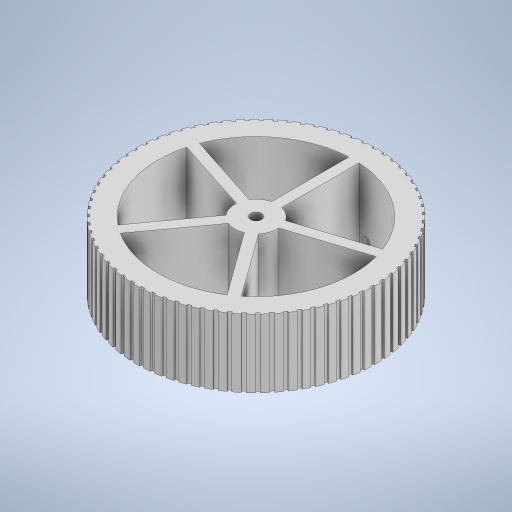
# Autodesk Inventor part: wheel
Saved by Autodesk Inventor 2023 (Build 270158000, 158)
## iProperties
Created: 2022-10-31
Part Number: wheel
Material: Generic
Document SubType Name: Modeling
Designer: neera
Density: 1 g/cm^3
Appearance: Default
Author: neera
Autodesk Inventor part; units mm, degrees
ref_plane "YZ Plane" through (0, 0, 0) normal (1, 0, 0) x (0, 1, 0)
ref_plane "XZ Plane" through (0, 0, 0) normal (0, 1, 0) x (-1, 0, 0)
ref_plane "XY Plane" through (0, 0, 0) normal (0, 0, 1) x (1, 0, 0)
sketch "Sketch1" plane through (0, 0, 0) normal (0, 1, 0) x (-1, 0, 0)
  circle A0 centre (0, 0) radius 70
  dimension "d0" = 140
  constraints: 1 centre point, 1 coincident
  measures "d0" diameter of A0
extrude "Extrusion1" add sketch "Sketch1" along normal blind 40
sketch "Sketch3" plane through (0, 40, 0) normal (0, 1, 0) x (1, 0, 0)
  circle A0 centre (0, 0) radius 57.5
  line L0 (0, 0) -> (57.5, 0) construction
  circle A1 centre (0, 0) radius 12.5
  line L1 (3, 12.1347) -> (3, 57.4217)
  line L2 (-3, 12.1347) -> (-3, 57.4217)
  line L3 (-10.6137, 6.603) -> (-53.6842, 20.5974)
  line L4 (-12.4678, 0.8966) -> (-55.5383, 14.8911)
  line L5 (-9.5596, -8.0538) -> (-36.1787, -44.6918)
  line L6 (-4.7055, -11.5805) -> (-31.3246, -48.2185)
  line L7 (4.7055, -11.5805) -> (31.3246, -48.2185)
  line L8 (9.5596, -8.0538) -> (36.1787, -44.6918)
  line L9 (12.4678, 0.8966) -> (55.5383, 14.8911)
  line L10 (10.6137, 6.603) -> (53.6842, 20.5974)
  point P0 (53.6842, 20.5974)
  dimension "d6" = 115
  dimension "d8" = 25
  dimension "d9" = 3
  dimension "d10" = 3
  dimension "d13" = 360
  constraints: 22 end point, 4 point on circle, 2 centre point, 2 coincident, 2 vertical, 1 horizontal, 31 other
  measures "d6" diameter of A0
  measures "d8" diameter of A1
  measures "d9" horizontal distance of point (0, 0) L1.start
  measures "d10" horizontal distance of point (0, 0) L2.start
extrude "Extrusion3" cut sketch "Sketch3" against normal blind 40 contours A0 L8 A1 L9 | L10 A1 L1 A0 | A0 L6 A1 L7 | L2 A1 L3 A0 | A0 L4 A1 L5
sketch "Sketch5" plane through (0, 0, 0) normal (0, -1, 0) x (1, 0, 0)
  arc A0 (-3.15, 0) -> (3.15, 0) centre (0, 0) ccw
  line L0 (3.15, 0) -> (12.5, 0)
  arc A1 (12.4678, -0.8966) -> (9.5596, 8.0538) centre (0, 0) ccw projected
  arc A2 (-1.695, 2.6551) -> (1.695, 2.6551) centre (0, 0) ccw projected
  line L1 (-3.15, 0) -> (-12.5073, 0)
  arc A3 (-12.5073, 0) -> (12.5, 0) centre (-0.0036, 0) ccw
  constraints: 6 point on circle, 4 end point, 2 centre point, 2 point on line, 1 coincident, 1 horizontal
extrude "Extrusion5" cut sketch "Sketch5" against normal blind 5
sketch "Sketch6" plane through (0, 0, 0) normal (0, -1, 0) x (1, 0, 0)
  circle A0 centre (0, 0) radius 3.15
  constraints: 1 centre point, 1 coincident
extrude "Extrusion6" cut sketch "Sketch6" against normal blind 40
sketch "Sketch7" plane through (12.5, 0, 0) normal (0, 0, -1) x (-1, 0, 0)
  circle A0 centre (4.675, 2.5) radius 1.5
  line L0 (9.35, 0) -> (9.35, 5) projected
  circle A1 centre (20.325, 2.5) radius 1.5
  line L1 (15.65, 0) -> (15.65, 5) projected
  line L2 (25, 5) -> (15.65, 5) projected
  line L3 (9.35, 5) -> (0, 5) projected
  point P0 (12.5, 0)
  point P1 (9.35, 2.5)
  point P2 (15.65, 2.5)
  point P3 (20.325, 5)
  point P4 (4.675, 5)
  dimension "d25" = 3
  dimension "d26" = 4.675
  dimension "d27" = 3
  dimension "d28" = 4.675
  dimension "d29" = 2.5
  dimension "d30" = 2.5
  constraints: 4 midpoint, 2 centre point
  measures "d25" diameter of A0
  measures "d26" distance of point (9.35, 2.5) A0.centre
  measures "d27" diameter of A1
  measures "d28" distance of point (15.65, 2.5) A1.centre
  measures "d29" distance of point (20.325, 5) A1.centre
  measures "d30" distance of point (4.675, 5) A0.centre
extrude "Extrusion7" cut sketch "Sketch7" against normal blind 4.5
sketch "Sketch8" plane through (0, 0, 0) normal (0, -1, 0) x (1, 0, 0)
  line L0 (6.325, 0) -> (6.325, 4.5) projected
  line L1 (9.325, 0) -> (9.325, 4.5) projected
  line L2 (6.325, 3) -> (9.325, 3)
  line L3 (9.325, 3) -> (9.325, 4.5)
  line L4 (9.325, 4.5) -> (6.325, 4.5)
  line L5 (6.325, 4.5) -> (6.325, 3)
  line L6 (-9.325, 0) -> (-9.325, 4.5) projected
  line L7 (-6.325, 0) -> (-6.325, 4.5) projected
  line L8 (-9.325, 3) -> (-6.325, 3)
  line L9 (-6.325, 3) -> (-6.325, 4.5)
  line L10 (-6.325, 4.5) -> (-9.325, 4.5)
  line L11 (-9.325, 4.5) -> (-9.325, 3)
  line L12 (-12.5, 0) -> (-3.15, 0) projected
  line L13 (3.15, 0) -> (12.5, 0) projected
  point P0 (0, 0)
  point P1 (-7.825, 0)
  point P2 (-7.825, 3)
  point P3 (7.825, 0)
  point P4 (7.825, 4.5)
  dimension "d33" = 3
  dimension "d34" = 4.5
  constraints: 16 end point, 6 point on line, 4 midpoint, 4 parallel, 2 horizontal, 2 perpendicular
  measures "d33" distance of point (-7.825, 0) point (-7.825, 3)
  measures "d34" distance of point (7.825, 0) point (7.825, 4.5)
extrude "Extrusion8" cut sketch "Sketch8" against normal blind 6 contours L0 L4 L1 L2 | L6 L10 L7 L8
sketch "Sketch9" plane through (0, 0, 0) normal (0, -1, 0) x (1, 0, 0)
  line L0 (1, -71) -> (-1, -71)
  line L1 (-1, -71) -> (-1, -69)
  line L2 (-1, -69) -> (1, -69)
  line L3 (1, -69) -> (1, -71)
  circle A0 centre (0, 0) radius 70 projected
  line L4 (1, -71) -> (-1, -69) construction
  line L5 (-1, -71) -> (1, -69) construction
  line L6 (4.7773, -68.8417) -> (6.7703, -68.6743)
  line L7 (6.7703, -68.6743) -> (6.9376, -70.6673)
  line L8 (4.9446, -70.8347) -> (4.7773, -68.8417)
  line L9 (6.9376, -70.6673) -> (4.9446, -70.8347)
  line L10 (10.521, -68.2005) -> (12.493, -67.867)
  line L11 (12.493, -67.867) -> (12.8266, -69.8389)
  line L12 (10.8546, -70.1725) -> (10.521, -68.2005)
  line L13 (12.8266, -69.8389) -> (10.8546, -70.1725)
  line L14 (16.191, -67.0809) -> (18.1282, -66.5835)
  line L15 (18.1282, -66.5835) -> (18.6256, -68.5207)
  line L16 (16.6884, -69.0181) -> (16.191, -67.0809)
  line L17 (18.6256, -68.5207) -> (16.6884, -69.0181)
  line L18 (21.7474, -65.4908) -> (23.6362, -64.8331)
  line L19 (23.6362, -64.8331) -> (24.2939, -66.7219)
  line L20 (22.4052, -67.3796) -> (21.7474, -65.4908)
  line L21 (24.2939, -66.7219) -> (22.4052, -67.3796)
  line L22 (27.1513, -63.4414) -> (28.9784, -62.6279)
  line L23 (28.9784, -62.6279) -> (29.7918, -64.455)
  line L24 (27.9648, -65.2685) -> (27.1513, -63.4414)
  line L25 (29.7918, -64.455) -> (27.9648, -65.2685)
  line L26 (32.3647, -60.9469) -> (34.1173, -59.9834)
  line L27 (34.1173, -59.9834) -> (35.0808, -61.736)
  line L28 (33.3282, -62.6995) -> (32.3647, -60.9469)
  line L29 (35.0808, -61.736) -> (33.3282, -62.6995)
  line L30 (37.3511, -58.025) -> (39.0169, -56.9182)
  line L31 (39.0169, -56.9182) -> (40.1237, -58.584)
  line L32 (38.4579, -59.6908) -> (37.3511, -58.025)
  line L33 (40.1237, -58.584) -> (38.4579, -59.6908)
  line L34 (42.0755, -54.696) -> (43.6429, -53.4537)
  line L35 (43.6429, -53.4537) -> (44.8852, -55.0211)
  line L36 (43.3178, -56.2634) -> (42.0755, -54.696)
  line L37 (44.8852, -55.0211) -> (43.3178, -56.2634)
  line L38 (46.5048, -50.9834) -> (47.9627, -49.6143)
  line L39 (47.9627, -49.6143) -> (49.3318, -51.0722)
  line L40 (47.8739, -52.4413) -> (46.5048, -50.9834)
  line L41 (49.3318, -51.0722) -> (47.8739, -52.4413)
  line L42 (50.6079, -46.9132) -> (51.9461, -45.4269)
  line L43 (51.9461, -45.4269) -> (53.4324, -46.7651)
  line L44 (52.0942, -48.2514) -> (50.6079, -46.9132)
  line L45 (53.4324, -46.7651) -> (52.0942, -48.2514)
  line L46 (54.356, -42.5139) -> (55.5652, -40.9208)
  line L47 (55.5652, -40.9208) -> (57.1582, -42.13)
  line L48 (55.949, -43.7231) -> (54.356, -42.5139)
  line L49 (57.1582, -42.13) -> (55.949, -43.7231)
  line L50 (57.7228, -37.8164) -> (58.7945, -36.1277)
  line L51 (58.7945, -36.1277) -> (60.4831, -37.1994)
  line L52 (59.4115, -38.888) -> (57.7228, -37.8164)
  line L53 (60.4831, -37.1994) -> (59.4115, -38.888)
  line L54 (60.6848, -32.8536) -> (61.6113, -31.0812)
  line L55 (61.6113, -31.0812) -> (63.3838, -32.0078)
  line L56 (62.4572, -33.7802) -> (60.6848, -32.8536)
  line L57 (63.3838, -32.0078) -> (62.4572, -33.7802)
  line L58 (63.221, -27.6604) -> (63.9961, -25.8167)
  line L59 (63.9961, -25.8167) -> (65.8398, -26.5917)
  line L60 (65.0648, -28.4355) -> (63.221, -27.6604)
  line L61 (65.8398, -26.5917) -> (65.0648, -28.4355)
  line L62 (65.3139, -22.2732) -> (65.9319, -20.3711)
  line L63 (65.9319, -20.3711) -> (67.834, -20.9892)
  line L64 (67.216, -22.8913) -> (65.3139, -22.2732)
  line L65 (67.834, -20.9892) -> (67.216, -22.8913)
  line L66 (66.9486, -16.7298) -> (67.4053, -14.7826)
  line L67 (67.4053, -14.7826) -> (69.3525, -15.2393)
  line L68 (68.8958, -17.1865) -> (66.9486, -16.7298)
  line L69 (69.3525, -15.2393) -> (68.8958, -17.1865)
  line L70 (68.1137, -11.069) -> (68.4059, -9.0905)
  line L71 (68.4059, -9.0905) -> (70.3844, -9.3826)
  line L72 (70.0923, -11.3612) -> (68.1137, -11.069)
  line L73 (70.3844, -9.3826) -> (70.0923, -11.3612)
  line L74 (68.8011, -5.3306) -> (68.9266, -3.3345)
  line L75 (68.9266, -3.3345) -> (70.9227, -3.4601)
  line L76 (70.7971, -5.4562) -> (68.8011, -5.3306)
  line L77 (70.9227, -3.4601) -> (70.7971, -5.4562)
  line L78 (69.0058, 0.4452) -> (68.9639, 2.4448)
  line L79 (68.9639, 2.4448) -> (70.9635, 2.4867)
  line L80 (71.0054, 0.4871) -> (69.0058, 0.4452)
  line L81 (70.9635, 2.4867) -> (71.0054, 0.4871)
  line L82 (68.7265, 6.2179) -> (68.5175, 8.207)
  line L83 (68.5175, 8.207) -> (70.5065, 8.416)
  line L84 (70.7156, 6.427) -> (68.7265, 6.2179)
  line L85 (70.5065, 8.416) -> (70.7156, 6.427)
  line L86 (67.9652, 11.947) -> (67.5904, 13.9116)
  line L87 (67.5904, 13.9116) -> (69.555, 14.2864)
  line L88 (69.9298, 12.3218) -> (67.9652, 11.947)
  line L89 (69.555, 14.2864) -> (69.9298, 12.3218)
  line L90 (66.7271, 17.5923) -> (66.1893, 19.5186)
  line L91 (66.1893, 19.5186) -> (68.1156, 20.0565)
  line L92 (68.6535, 18.1301) -> (66.7271, 17.5923)
  line L93 (68.1156, 20.0565) -> (68.6535, 18.1301)
  line L94 (65.021, 23.1142) -> (64.3239, 24.9888)
  line L95 (64.3239, 24.9888) -> (66.1984, 25.6859)
  line L96 (66.8956, 23.8113) -> (65.021, 23.1142)
  line L97 (66.1984, 25.6859) -> (66.8956, 23.8113)
  line L98 (62.8588, 28.4739) -> (62.0073, 30.2836)
  line L99 (62.0073, 30.2836) -> (63.8169, 31.1352)
  line L100 (64.6685, 29.3255) -> (62.8588, 28.4739)
  line L101 (63.8169, 31.1352) -> (64.6685, 29.3255)
  line L102 (60.2558, 33.634) -> (59.2558, 35.366)
  line L103 (59.2558, 35.366) -> (60.9878, 36.366)
  line L104 (61.9878, 34.634) -> (60.2558, 33.634)
  line L105 (60.9878, 36.366) -> (61.9878, 34.634)
  line L106 (57.23, 38.5581) -> (56.0886, 40.2004)
  line L107 (56.0886, 40.2004) -> (57.7309, 41.3418)
  line L108 (58.8723, 39.6995) -> (57.23, 38.5581)
  line L109 (57.7309, 41.3418) -> (58.8723, 39.6995)
  line L110 (53.8028, 43.2117) -> (52.528, 44.7528)
  line L111 (52.528, 44.7528) -> (54.069, 46.0276)
  line L112 (55.3439, 44.4866) -> (53.8028, 43.2117)
  line L113 (54.069, 46.0276) -> (55.3439, 44.4866)
  line L114 (49.9983, 47.5623) -> (48.599, 48.9912)
  line L115 (48.599, 48.9912) -> (50.0279, 50.3906)
  line L116 (51.4272, 48.9616) -> (49.9983, 47.5623)
  line L117 (50.0279, 50.3906) -> (51.4272, 48.9616)
  line L118 (45.843, 51.5792) -> (44.329, 52.8861)
  line L119 (44.329, 52.8861) -> (45.6359, 54.4001)
  line L120 (47.1499, 53.0932) -> (45.843, 51.5792)
  line L121 (45.6359, 54.4001) -> (47.1499, 53.0932)
  line L122 (41.3662, 55.2344) -> (39.7482, 56.41)
  line L123 (39.7482, 56.41) -> (40.9237, 58.028)
  line L124 (42.5418, 56.8524) -> (41.3662, 55.2344)
  line L125 (40.9237, 58.028) -> (42.5418, 56.8524)
  line L126 (36.5992, 58.5021) -> (34.8885, 59.5382)
  line L127 (34.8885, 59.5382) -> (35.9246, 61.2489)
  line L128 (37.6353, 60.2128) -> (36.5992, 58.5021)
  line L129 (35.9246, 61.2489) -> (37.6353, 60.2128)
  line L130 (31.5755, 61.3595) -> (29.7841, 62.2487)
  line L131 (29.7841, 62.2487) -> (30.6734, 64.0402)
  line L132 (32.4648, 63.1509) -> (31.5755, 61.3595)
  line L133 (30.6734, 64.0402) -> (32.4648, 63.1509)
  line L134 (26.3304, 63.7865) -> (24.4708, 64.5227)
  line L135 (24.4708, 64.5227) -> (25.2071, 66.3823)
  line L136 (27.0666, 65.646) -> (26.3304, 63.7865)
  line L137 (25.2071, 66.3823) -> (27.0666, 65.646)
  line L138 (20.9005, 65.766) -> (18.9859, 66.3441)
  line L139 (18.9859, 66.3441) -> (19.5639, 68.2587)
  line L140 (21.4786, 67.6807) -> (20.9005, 65.766)
  line L141 (19.5639, 68.2587) -> (21.4786, 67.6807)
  line L142 (15.3241, 67.2843) -> (13.3678, 67.7001)
  line L143 (13.3678, 67.7001) -> (13.7836, 69.6564)
  line L144 (15.7399, 69.2406) -> (15.3241, 67.2843)
  line L145 (13.7836, 69.6564) -> (15.7399, 69.2406)
  line L146 (9.6401, 68.3306) -> (7.6559, 68.5812)
  line L147 (7.6559, 68.5812) -> (7.9065, 70.5655)
  line L148 (9.8908, 70.3148) -> (9.6401, 68.3306)
  line L149 (7.9065, 70.5655) -> (9.8908, 70.3148)
  line L150 (3.8885, 68.8976) -> (1.8903, 68.9814)
  line L151 (1.8903, 68.9814) -> (1.974, 70.9796)
  line L152 (3.9723, 70.8958) -> (3.8885, 68.8976)
  line L153 (1.974, 70.9796) -> (3.9723, 70.8958)
  line L154 (-1.8903, 68.9814) -> (-3.8885, 68.8976)
  line L155 (-3.8885, 68.8976) -> (-3.9723, 70.8958)
  line L156 (-1.974, 70.9796) -> (-1.8903, 68.9814)
  line L157 (-3.9723, 70.8958) -> (-1.974, 70.9796)
  line L158 (-7.6559, 68.5812) -> (-9.6401, 68.3306)
  line L159 (-9.6401, 68.3306) -> (-9.8908, 70.3148)
  line L160 (-7.9065, 70.5655) -> (-7.6559, 68.5812)
  line L161 (-9.8908, 70.3148) -> (-7.9065, 70.5655)
  line L162 (-13.3678, 67.7001) -> (-15.3241, 67.2843)
  line L163 (-15.3241, 67.2843) -> (-15.7399, 69.2406)
  line L164 (-13.7836, 69.6564) -> (-13.3678, 67.7001)
  line L165 (-15.7399, 69.2406) -> (-13.7836, 69.6564)
  line L166 (-18.9859, 66.3441) -> (-20.9005, 65.766)
  line L167 (-20.9005, 65.766) -> (-21.4786, 67.6807)
  line L168 (-19.5639, 68.2587) -> (-18.9859, 66.3441)
  line L169 (-21.4786, 67.6807) -> (-19.5639, 68.2587)
  line L170 (-24.4708, 64.5227) -> (-26.3304, 63.7865)
  line L171 (-26.3304, 63.7865) -> (-27.0666, 65.646)
  line L172 (-25.2071, 66.3823) -> (-24.4708, 64.5227)
  line L173 (-27.0666, 65.646) -> (-25.2071, 66.3823)
  line L174 (-29.7841, 62.2487) -> (-31.5755, 61.3595)
  line L175 (-31.5755, 61.3595) -> (-32.4648, 63.1509)
  line L176 (-30.6734, 64.0402) -> (-29.7841, 62.2487)
  line L177 (-32.4648, 63.1509) -> (-30.6734, 64.0402)
  line L178 (-34.8885, 59.5382) -> (-36.5992, 58.5021)
  line L179 (-36.5992, 58.5021) -> (-37.6353, 60.2128)
  line L180 (-35.9246, 61.2489) -> (-34.8885, 59.5382)
  line L181 (-37.6353, 60.2128) -> (-35.9246, 61.2489)
  line L182 (-39.7482, 56.41) -> (-41.3662, 55.2344)
  line L183 (-41.3662, 55.2344) -> (-42.5418, 56.8524)
  line L184 (-40.9237, 58.028) -> (-39.7482, 56.41)
  line L185 (-42.5418, 56.8524) -> (-40.9237, 58.028)
  line L186 (-44.329, 52.8861) -> (-45.843, 51.5792)
  line L187 (-45.843, 51.5792) -> (-47.1499, 53.0932)
  line L188 (-45.6359, 54.4001) -> (-44.329, 52.8861)
  line L189 (-47.1499, 53.0932) -> (-45.6359, 54.4001)
  line L190 (-48.599, 48.9912) -> (-49.9983, 47.5623)
  line L191 (-49.9983, 47.5623) -> (-51.4272, 48.9616)
  line L192 (-50.0279, 50.3906) -> (-48.599, 48.9912)
  line L193 (-51.4272, 48.9616) -> (-50.0279, 50.3906)
  line L194 (-52.528, 44.7528) -> (-53.8028, 43.2117)
  line L195 (-53.8028, 43.2117) -> (-55.3439, 44.4866)
  line L196 (-54.069, 46.0276) -> (-52.528, 44.7528)
  line L197 (-55.3439, 44.4866) -> (-54.069, 46.0276)
  line L198 (-56.0886, 40.2004) -> (-57.23, 38.5581)
  line L199 (-57.23, 38.5581) -> (-58.8723, 39.6995)
  line L200 (-57.7309, 41.3418) -> (-56.0886, 40.2004)
  line L201 (-58.8723, 39.6995) -> (-57.7309, 41.3418)
  line L202 (-59.2558, 35.366) -> (-60.2558, 33.634)
  line L203 (-60.2558, 33.634) -> (-61.9878, 34.634)
  line L204 (-60.9878, 36.366) -> (-59.2558, 35.366)
  line L205 (-61.9878, 34.634) -> (-60.9878, 36.366)
  line L206 (-62.0073, 30.2836) -> (-62.8588, 28.4739)
  line L207 (-62.8588, 28.4739) -> (-64.6685, 29.3255)
  line L208 (-63.8169, 31.1352) -> (-62.0073, 30.2836)
  line L209 (-64.6685, 29.3255) -> (-63.8169, 31.1352)
  line L210 (-64.3239, 24.9888) -> (-65.021, 23.1142)
  line L211 (-65.021, 23.1142) -> (-66.8956, 23.8113)
  line L212 (-66.1984, 25.6859) -> (-64.3239, 24.9888)
  line L213 (-66.8956, 23.8113) -> (-66.1984, 25.6859)
  line L214 (-66.1893, 19.5186) -> (-66.7271, 17.5923)
  line L215 (-66.7271, 17.5923) -> (-68.6535, 18.1301)
  line L216 (-68.1156, 20.0565) -> (-66.1893, 19.5186)
  line L217 (-68.6535, 18.1301) -> (-68.1156, 20.0565)
  line L218 (-67.5904, 13.9116) -> (-67.9652, 11.947)
  line L219 (-67.9652, 11.947) -> (-69.9298, 12.3218)
  line L220 (-69.555, 14.2864) -> (-67.5904, 13.9116)
  line L221 (-69.9298, 12.3218) -> (-69.555, 14.2864)
  line L222 (-68.5175, 8.207) -> (-68.7265, 6.2179)
  line L223 (-68.7265, 6.2179) -> (-70.7156, 6.427)
  line L224 (-70.5065, 8.416) -> (-68.5175, 8.207)
  line L225 (-70.7156, 6.427) -> (-70.5065, 8.416)
  line L226 (-68.9639, 2.4448) -> (-69.0058, 0.4452)
  line L227 (-69.0058, 0.4452) -> (-71.0054, 0.4871)
  line L228 (-70.9635, 2.4867) -> (-68.9639, 2.4448)
  line L229 (-71.0054, 0.4871) -> (-70.9635, 2.4867)
  line L230 (-68.9266, -3.3345) -> (-68.8011, -5.3306)
  line L231 (-68.8011, -5.3306) -> (-70.7971, -5.4562)
  line L232 (-70.9227, -3.4601) -> (-68.9266, -3.3345)
  line L233 (-70.7971, -5.4562) -> (-70.9227, -3.4601)
  line L234 (-68.4059, -9.0905) -> (-68.1137, -11.069)
  line L235 (-68.1137, -11.069) -> (-70.0923, -11.3612)
  line L236 (-70.3844, -9.3826) -> (-68.4059, -9.0905)
  line L237 (-70.0923, -11.3612) -> (-70.3844, -9.3826)
  line L238 (-67.4053, -14.7826) -> (-66.9486, -16.7298)
  line L239 (-66.9486, -16.7298) -> (-68.8958, -17.1865)
  line L240 (-69.3525, -15.2393) -> (-67.4053, -14.7826)
  line L241 (-68.8958, -17.1865) -> (-69.3525, -15.2393)
  line L242 (-65.9319, -20.3711) -> (-65.3139, -22.2732)
  line L243 (-65.3139, -22.2732) -> (-67.216, -22.8913)
  line L244 (-67.834, -20.9892) -> (-65.9319, -20.3711)
  line L245 (-67.216, -22.8913) -> (-67.834, -20.9892)
  line L246 (-63.9961, -25.8167) -> (-63.221, -27.6604)
  line L247 (-63.221, -27.6604) -> (-65.0648, -28.4355)
  line L248 (-65.8398, -26.5917) -> (-63.9961, -25.8167)
  line L249 (-65.0648, -28.4355) -> (-65.8398, -26.5917)
  line L250 (-61.6113, -31.0812) -> (-60.6848, -32.8536)
  line L251 (-60.6848, -32.8536) -> (-62.4572, -33.7802)
  line L252 (-63.3838, -32.0078) -> (-61.6113, -31.0812)
  line L253 (-62.4572, -33.7802) -> (-63.3838, -32.0078)
  line L254 (-58.7945, -36.1277) -> (-57.7228, -37.8164)
  line L255 (-57.7228, -37.8164) -> (-59.4115, -38.888)
  line L256 (-60.4831, -37.1994) -> (-58.7945, -36.1277)
  line L257 (-59.4115, -38.888) -> (-60.4831, -37.1994)
  line L258 (-55.5652, -40.9208) -> (-54.356, -42.5139)
  line L259 (-54.356, -42.5139) -> (-55.949, -43.7231)
  line L260 (-57.1582, -42.13) -> (-55.5652, -40.9208)
  line L261 (-55.949, -43.7231) -> (-57.1582, -42.13)
  line L262 (-51.9461, -45.4269) -> (-50.6079, -46.9132)
  line L263 (-50.6079, -46.9132) -> (-52.0942, -48.2514)
  line L264 (-53.4324, -46.7651) -> (-51.9461, -45.4269)
  line L265 (-52.0942, -48.2514) -> (-53.4324, -46.7651)
  line L266 (-47.9627, -49.6143) -> (-46.5048, -50.9834)
  line L267 (-46.5048, -50.9834) -> (-47.8739, -52.4413)
  line L268 (-49.3318, -51.0722) -> (-47.9627, -49.6143)
  line L269 (-47.8739, -52.4413) -> (-49.3318, -51.0722)
  line L270 (-43.6429, -53.4537) -> (-42.0755, -54.696)
  line L271 (-42.0755, -54.696) -> (-43.3178, -56.2634)
  line L272 (-44.8852, -55.0211) -> (-43.6429, -53.4537)
  line L273 (-43.3178, -56.2634) -> (-44.8852, -55.0211)
  line L274 (-39.0169, -56.9182) -> (-37.3511, -58.025)
  line L275 (-37.3511, -58.025) -> (-38.4579, -59.6908)
  line L276 (-40.1237, -58.584) -> (-39.0169, -56.9182)
  line L277 (-38.4579, -59.6908) -> (-40.1237, -58.584)
  line L278 (-34.1173, -59.9834) -> (-32.3647, -60.9469)
  line L279 (-32.3647, -60.9469) -> (-33.3282, -62.6995)
  line L280 (-35.0808, -61.736) -> (-34.1173, -59.9834)
  line L281 (-33.3282, -62.6995) -> (-35.0808, -61.736)
  line L282 (-28.9784, -62.6279) -> (-27.1513, -63.4414)
  line L283 (-27.1513, -63.4414) -> (-27.9648, -65.2685)
  line L284 (-29.7918, -64.455) -> (-28.9784, -62.6279)
  line L285 (-27.9648, -65.2685) -> (-29.7918, -64.455)
  line L286 (-23.6362, -64.8331) -> (-21.7474, -65.4908)
  line L287 (-21.7474, -65.4908) -> (-22.4052, -67.3796)
  line L288 (-24.2939, -66.7219) -> (-23.6362, -64.8331)
  line L289 (-22.4052, -67.3796) -> (-24.2939, -66.7219)
  line L290 (-18.1282, -66.5835) -> (-16.191, -67.0809)
  line L291 (-16.191, -67.0809) -> (-16.6884, -69.0181)
  line L292 (-18.6256, -68.5207) -> (-18.1282, -66.5835)
  line L293 (-16.6884, -69.0181) -> (-18.6256, -68.5207)
  line L294 (-12.493, -67.867) -> (-10.521, -68.2005)
  line L295 (-10.521, -68.2005) -> (-10.8546, -70.1725)
  line L296 (-12.8266, -69.8389) -> (-12.493, -67.867)
  line L297 (-10.8546, -70.1725) -> (-12.8266, -69.8389)
  line L298 (-6.7703, -68.6743) -> (-4.7773, -68.8417)
  line L299 (-4.7773, -68.8417) -> (-4.9446, -70.8347)
  line L300 (-6.9376, -70.6673) -> (-6.7703, -68.6743)
  line L301 (-4.9446, -70.8347) -> (-6.9376, -70.6673)
  point P0 (0, -70)
  point P1 (-46.4918, 52.3308)
  point P2 (-44.9778, 53.6377)
  point P3 (-41.9498, 56.0376)
  point P4 (-40.3318, 57.2132)
  point P5 (-37.1136, 59.3514)
  point P6 (-35.4028, 60.3874)
  point P7 (-21.1875, 66.7165)
  point P8 (-19.2728, 67.2946)
  point P9 (-3.9301, 69.8896)
  point P10 (-1.9319, 69.9733)
  point P11 (1.9319, 69.9733)
  point P12 (3.9301, 69.8896)
  point P13 (7.7803, 69.5663)
  point P14 (9.7645, 69.3156)
  point P15 (13.5742, 68.6713)
  point P16 (15.5305, 68.2554)
  point P17 (35.4028, 60.3874)
  point P18 (37.1136, 59.3514)
  point P19 (44.9778, 53.6377)
  point P20 (46.4918, 52.3308)
  dimension "d37" = 2
  dimension "d38" = 2
  dimension "d41" = 360
  constraints: 604 end point, 2 midpoint, 2 parallel, 1 horizontal, 1 perpendicular, 603 other
  measures "d37" distance of L1.end L2.end
  measures "d38" distance of L0.end L1.end
extrude "Extrusion9" cut sketch "Sketch9" against normal blind 40 contours L0 L1 A0 L3 | A0 L1 L2 L3 | L8 L6 L7 A0 | A0 L7 L9 L8 | L299 L301 L300 A0 | A0 L300 L298 L299 | L12 L10 L11 A0 | A0 L11 L13 L12 | L295 L297 L296 A0 | A0 L296 L294 L295 | L16 L14 L15 A0 | A0 L15 L17 L16 | L291 L293 L292 A0 | A0 L292 L290 L291 | L20 L18 L19 A0 | A0 L19 L21 L20 | L287 L289 L288 A0 | A0 L288 L286 L287 | L24 L22 L23 A0 | A0 L23 L25 L24 | L283 L285 L284 A0 | A0 L284 L282 L283 | L28 L26 L27 A0 | A0 L27 L29 L28 | L279 L281 L280 A0 | A0 L280 L278 L279 | L32 L30 L31 A0 | A0 L31 L33 L32 | L275 L277 L276 A0 | A0 L276 L274 L275 | L36 L34 L35 A0 | A0 L35 L37 L36 | L271 L273 L272 A0 | A0 L272 L270 L271 | L40 L38 L39 A0 | A0 L39 L41 L40 | L267 L269 L268 A0 | A0 L268 L266 L267 | L44 L42 L43 A0 | A0 L43 L45 L44 | L263 L265 L264 A0 | A0 L264 L262 L263 | L48 L46 L47 A0 | A0 L47 L49 L48 | L259 L261 L260 A0 | A0 L260 L258 L259 | L52 L50 L51 A0 | A0 L51 L53 L52 | L255 L257 L256 A0 | A0 L256 L254 L255 | L56 L54 L55 A0 | A0 L55 L57 L56 | L251 L253 L252 A0 | A0 L252 L250 L251 | L60 L58 L59 A0 | A0 L59 L61 L60 | L247 L249 L248 A0 | A0 L248 L246 L247 | L64 L62 L63 A0 | A0 L63 L65 L64 | L243 L245 L244 A0 | A0 L244 L242 L243 | L68 L66 L67 A0 | A0 L67 L69 L68 | L239 L241 L240 A0 | A0 L240 L238 L239 | L72 L70 L71 A0 | A0 L71 L73 L72 | L235 L237 L236 A0 | A0 L236 L234 L235 | L76 L74 L75 A0 | A0 L75 L77 L76 | L231 L233 L232 A0 | A0 L232 L230 L231 | L227 L229 L228 A0 | A0 L228 L226 L227 | L80 L78 L79 A0 | A0 L79 L81 L80 | L223 L225 L224 A0 | A0 L224 L222 L223 | L84 L82 L83 A0 | A0 L83 L85 L84 | L219 L221 L220 A0 | A0 L220 L218 L219 | L88 L86 L87 A0 | A0 L87 L89 L88 | L215 L217 L216 A0 | A0 L216 L214 L215 | L92 L90 L91 A0 | A0 L91 L93 L92 | L211 L213 L212 A0 | A0 L212 L210 L211 | L96 L94 L95 A0 | A0 L95 L97 L96 | L207 L209 L208 A0 | A0 L208 L206 L207 | L100 L98 L99 A0 | A0 L99 L101 L100 | L203 L205 L204 A0 | A0 L204 L202 L203 | L104 L102 L103 A0 | A0 L103 L105 L104 | L199 L201 L200 A0 | A0 L200 L198 L199 | L108 L106 L107 A0 | A0 L107 L109 L108 | L195 L197 L196 A0 | A0 L196 L194 L195 | L112 L110 L111 A0 | A0 L111 L113 L112 | L191 L193 L192 A0 | A0 L192 L190 L191 | L116 L114 L115 A0 | A0 L115 L117 L116 | L187 L189 L188 A0 | A0 L188 L186 L187 | L120 L118 L119 A0 | A0 L119 L121 L120 | L183 L185 L184 A0 | A0 L184 L182 L183 | L124 L122 L123 A0 | A0 L123 L125 L124 | L179 L181 L180 A0 | A0 L180 L178 L179 | L128 L126 L127 A0 | A0 L127 L129 L128 | L175 L177 L176 A0 | A0 L176 L174 L175 | L132 L130 L131 A0 | A0 L131 L133 L132 | L171 L173 L172 A0 | A0 L172 L170 L171 | L136 L134 L135 A0 | A0 L135 L137 L136 | L167 L169 L168 A0 | A0 L168 L166 L167 | L140 L138 L139 A0 | A0 L139 L141 L140 | L163 L165 L164 A0 | A0 L164 L162 L163 | L144 L142 L143 A0 | A0 L143 L145 L144 | L159 L161 L160 A0 | A0 L160 L158 L159 | L148 L146 L147 A0 | A0 L147 L149 L148 | L155 L157 L156 A0 | A0 L156 L154 L155 | L152 L150 L151 A0 | A0 L151 L153 L152
sketch "Sketch10" plane through (12.5, 0, 0) normal (0, 0, -1) x (-1, 0, 0)
  circle A0 centre (4.675, 2.5) radius 2.5
  line L0 (9.35, 0) -> (9.35, 5) projected
  line L1 (9.35, 5) -> (0, 5) projected
  circle A1 centre (20.325, 2.5) radius 2.5
  line L2 (15.65, 0) -> (15.65, 5) projected
  line L3 (25, 5) -> (15.65, 5) projected
  point P0 (12.5, 0)
  point P1 (9.35, 2.5)
  point P2 (15.65, 2.5)
  point P3 (20.325, 5)
  dimension "d45" = 5
  dimension "d46" = 4.675
  dimension "d47" = 2.5
  dimension "d48" = 5
  dimension "d49" = 4.675
  dimension "d50" = 2.5
  constraints: 3 midpoint, 2 centre point
  measures "d45" diameter of A0
  measures "d46" distance of point (9.35, 2.5) A0.centre
  measures "d47" distance from line of L1 A0.centre
  measures "d48" diameter of A1
  measures "d49" distance of point (15.65, 2.5) A1.centre
  measures "d50" distance of point (20.325, 5) A1.centre
extrude "Extrusion10" cut sketch "Sketch10" along normal blind 80
body "Solid1"
